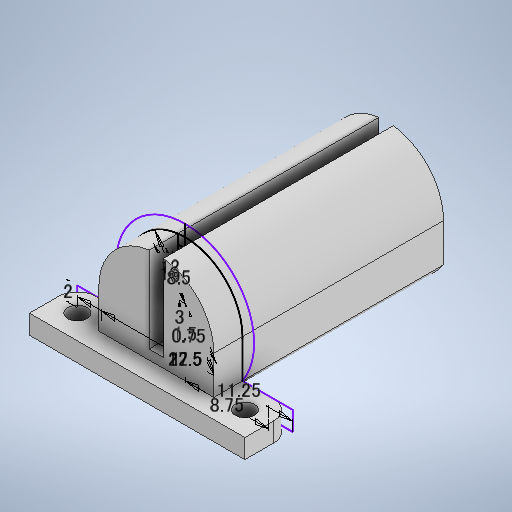
# Autodesk Inventor part: motor cover1
Saved by Autodesk Inventor 2025 (Build 290162000, 162)
## iProperties
Created: 2024-05-21
Part Number: motor cover1
Material: 一般
Document SubType Name: Modeling
Designer: Saigusa
Density: 1 g/cm^3
Appearance: 既定
Author: Saigusa
Autodesk Inventor part; units mm, degrees
ref_plane "YZ Plane" through (0, 0, 0) normal (1, 0, 0) x (0, 1, 0)
ref_plane "XZ Plane" through (0, 0, 0) normal (0, 1, 0) x (-1, 0, 0)
ref_plane "XY Plane" through (0, 0, 0) normal (0, 0, 1) x (1, 0, 0)
sketch "スケッチ1" plane through (0, 0, 0) normal (0, 0, 1) x (1, 0, 0)
  circle A0 centre (0, 0) radius 4.25
  circle A1 centre (0, 0) radius 4.5
  circle A2 centre (0, 0) radius 5
  line L0 (0, -5) -> (0, -6)
  line L1 (0, -6) -> (8.75, -6)
  line L2 (8.75, -6) -> (-8.75, -6)
  line L3 (0, -6) -> (11.25, -6)
  line L4 (11.25, -6) -> (-11.25, -6)
  line L5 (-11.25, -6) -> (-11.25, -4)
  line L6 (-11.25, -4) -> (11.25, -4)
  line L7 (11.25, -4) -> (11.25, -6)
  circle A3 centre (0, 0) radius 6
  line L8 (-6, 0) -> (-6, -4)
  line L9 (6, 0) -> (6, -4)
  circle A4 centre (0, 0) radius 7.2111
  line L10 (0, 0) -> (0, -3)
  line L11 (0, -3) -> (0, 7.2111)
  line L12 (0, -3) -> (0.75, -3)
  line L13 (0.75, -3) -> (-0.75, -3)
  line L14 (-0.75, -3) -> (-0.75, 5.9529)
  line L15 (0.75, -3) -> (0.75, 5.9529)
  point P0 (4.4721, -4)
  point P1 (-4.4721, -4)
  point P2 (4, -6)
  point P3 (-4, -6)
  point P4 (-0.75, 4.4371)
  point P5 (0.75, 4.4371)
  dimension "d2" = 10
  dimension "d0" = 8.5
  dimension "d1" = 9
  dimension "d3" = 1
  dimension "d4" = 8.75
  dimension "d5" = 17.5
  dimension "d6" = 11.25
  dimension "d7" = 22.5
  dimension "d8" = 2
  dimension "d9" = 12
  dimension "d18" = 3
  dimension "d19" = 0.75
  dimension "d20" = 1.5
  constraints: 32 end point, 8 perpendicular, 7 point on line, 6 point on circle, 5 coincident, 4 centre point, 2 tangent, 2 vertical, 1 parallel, 1 vertical alignment, 2 other
  measures "d0" diameter of A0
  measures "d1" diameter of A1
  measures "d3" distance of L0.start L0.end
  measures "d4" distance of L0.end L1.end
  measures "d5" distance of L1.end L2.end
  measures "d6" distance of L0.end L3.end
  measures "d7" distance of L3.end L4.end
  measures "d8" distance of L4.end L5.end
  measures "d9" diameter of A3
  measures "d18" distance of L10.start L10.end
  measures "d19" distance of L10.end L12.end
  measures "d20" distance of L12.end L13.end
extrude "押し出し1" add sketch "スケッチ1" along normal blind 5 contours L6 A1 A0 | A0 L6 | L6 A2 A1 | L6 A3 L0 A2 | A2 L0 A3 L6 | L6 A4 L1 A3 | A3 L2 A4 L6 | L6 L7 L3 L1 A4 | A4 L2 L4 L5 L6
extrude "押し出し2" add sketch "スケッチ1" along normal blind 3 contours A0 L6 L14 L13 L12 L15 | A0 L15 A1 L6 | L15 L12 L10 L11 A0 | A0 L11 A1 L15 | L6 A1 A0 | A0 L6 | L11 L10 L13 L14 A0 | A0 L14 A1 L11 | L15 A2 L6 A1 | A1 L11 A2 L15 | L6 A1 L14 A0 | L6 A2 A1 | A1 L14 A2 L11 | L15 A3 L6 A2 | A2 L11 A3 L15 | L6 A2 L14 A1 | L6 A3 L0 A2 | A2 L14 A3 L11 | L6 A3 L14 A2 | A2 L0 A3 L6 | A3 L9 L6 | L6 L8 A3
extrude "押し出し3" add sketch "スケッチ1" against normal blind 21 contours L15 A2 L6 A1 | A1 L11 A2 L15 | L6 A2 A1 | A1 L14 A2 L11 | L15 A3 L6 A2 | A2 L11 A3 L15 | L6 A2 L14 A1 | L6 A3 L0 A2 | A2 L14 A3 L11 | L6 A3 L14 A2 | A2 L0 A3 L6 | A3 L9 L6 | L6 A4 L1 A3 | A3 L2 A4 L6 | L6 L8 A3
extrude "押し出し4" cut sketch "スケッチ1" along normal blind 1.5 contours A0 L6 L14 L13 L12 L15 | A0 L15 A1 L6 | L15 L12 L10 L11 A0 | A0 L11 A1 L15 | L6 A1 A0 | A0 L6 | L11 L10 L13 L14 A0 | A0 L14 A1 L11 | L6 A1 L14 A0
extrude "押し出し5" cut sketch "スケッチ1" along normal blind 3 contours L15 L12 L10 L11 A0 | A0 L11 A1 L15 | L11 L10 L13 L14 A0 | A0 L14 A1 L11 | A1 L11 A2 L15 | A1 L14 A2 L11 | A2 L11 A3 L15 | A2 L14 A3 L11
extrude "押し出し6" cut sketch "スケッチ1" against normal blind 21 contours A1 L11 A2 L15 | A1 L14 A2 L11 | A2 L11 A3 L15 | A2 L14 A3 L11
sketch "スケッチ2" plane through (-11.25, -4, 5) normal (0, 1, 0) x (1, 0, 0)
  line L0 (22.5, 0) -> (0, 0) projected
  line L1 (0, 0) -> (0, 2.5)
  line L2 (0, 5) -> (0, 0) projected
  line L3 (0, 2.5) -> (22.5, 2.5)
  line L4 (22.5, 5) -> (22.5, 0) projected
  line L5 (22.5, 2.5) -> (20, 2.5)
  line L6 (20, 2.5) -> (2.5, 2.5)
  point P0 (11.25, 5)
  dimension "d25" = 2.5
  dimension "d26" = 17.5
  constraints: 8 end point, 2 midpoint, 2 point on line
  measures "d25" distance of L3.end L5.end
  measures "d26" distance of L5.end L6.end
hole "穴1" at (-8.75, -4, 2.5) at (8.75, -4, 2.5) direction (0, -1, 0) diameter 2 end through all
fillet "フィレット1" radius 2 2 edges at (-11.25, -5, 0) (11.25, -5, 0)
